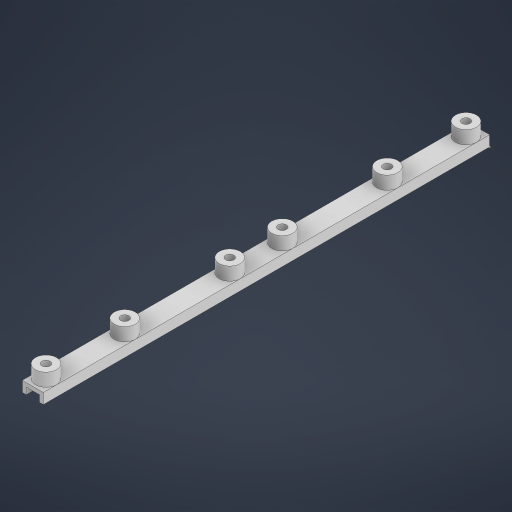
# Autodesk Inventor part: chassis_brace_jig
Saved by Autodesk Inventor 2024 (Build 280153000, 153)
## iProperties
Created: 2024-01-19
Part Number: chassis_brace_jig
Material: Generic
Document SubType Name: Modeling
Designer: avere
Density: 1 g/cm^3
Appearance: Default
Author: avere
Autodesk Inventor part; units mm, degrees
ref_plane "YZ Plane" through (0, 0, 0) normal (1, 0, 0) x (0, 1, 0)
ref_plane "XZ Plane" through (0, 0, 0) normal (0, 1, 0) x (-1, 0, 0)
ref_plane "XY Plane" through (0, 0, 0) normal (0, 0, 1) x (1, 0, 0)
sketch "Sketch1" plane through (0, 0, 0) normal (0, 0, 1) x (1, 0, 0)
  line L0 (3.175, 0) -> (3.175, 3.175)
  line L1 (3.175, 3.175) -> (-3.175, 3.175)
  line L2 (-3.175, 3.175) -> (-3.175, 0)
  line L3 (5.08, 0) -> (5.08, 5.08)
  line L4 (5.08, 5.08) -> (-5.08, 5.08)
  line L5 (-5.08, 5.08) -> (-5.08, 0)
  line L6 (-5.08, 0) -> (-3.175, 0)
  line L7 (3.175, 0) -> (5.08, 0)
  point P0 (0, 0)
  dimension "d0" = 6.35
  dimension "d1" = 3.175
  dimension "d2" = 10.16
  dimension "d3" = 5.08
  constraints: 16 end point, 4 parallel, 2 horizontal, 2 perpendicular
  measures "d0" distance of L1.end L0.end
  measures "d1" distance of L0.end L0.start
  measures "d2" distance of L4.end L3.end
  measures "d3" distance of L3.end L3.start
extrude "Extrusion1" add sketch "Sketch1" along normal blind 215.9
sketch "Sketch2" plane through (-5.08, 5.08, 0) normal (0, 1, 0) x (1, 0, 0)
  circle A0 centre (5.08, -6.35) radius 1.985
  circle A1 centre (5.08, -209.55) radius 1.985
  circle A2 centre (5.08, -44.45) radius 1.985
  circle A3 centre (5.08, -171.45) radius 1.985
  circle A4 centre (5.08, -95.25) radius 1.985
  circle A5 centre (5.08, -120.65) radius 1.985
  point P0 (5.08, 0)
  dimension "d6" = 3.97
  dimension "d7" = 3.97
  dimension "d8" = 3.97
  dimension "d9" = 3.97
  dimension "d10" = 3.97
  dimension "d11" = 3.97
  constraints: 6 centre point
  measures "d6" diameter of A0
  measures "d7" diameter of A1
  measures "d8" diameter of A2
  measures "d9" diameter of A3
  measures "d10" diameter of A4
  measures "d11" diameter of A5
extrude "Extrusion2" cut sketch "Sketch2" against normal blind 215.9
sketch "Sketch3" plane through (5.08, 0, 0) normal (1, 0, 0) x (0, 0, -1)
  point P0 (0, 0)
sketch "Sketch4" plane through (-5.08, 5.08, 0) normal (0, 1, 0) x (1, 0, 0)
  circle A0 centre (5.08, -6.35) radius 1.985 projected
  circle A1 centre (5.08, -44.45) radius 1.985 projected
  circle A2 centre (5.08, -95.25) radius 1.985 projected
  circle A3 centre (5.08, -120.65) radius 1.985 projected
  circle A4 centre (5.08, -171.45) radius 1.985 projected
  circle A5 centre (5.08, -6.35) radius 5.08
  circle A6 centre (5.08, -44.45) radius 5.08
  line L0 (0, 0) -> (0, -215.9) projected
  circle A7 centre (5.08, -95.25) radius 5.08
  circle A8 centre (5.08, -120.65) radius 5.08
  circle A9 centre (5.08, -171.45) radius 5.08
  circle A10 centre (5.08, -209.55) radius 1.985 projected
  circle A11 centre (5.08, -209.55) radius 5.08
  point P0 (5.08, 0)
  constraints: 6 centre point, 6 coincident, 2 tangent
extrude "Extrusion3" add sketch "Sketch4" along normal blind 6.35
body "Solid1"
